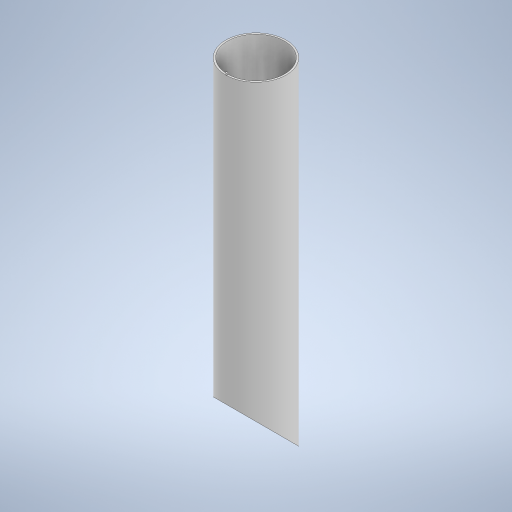
# Autodesk Inventor part: Feul_Intake
Saved by Autodesk Inventor 2024.3 (Build 283343000, 343)
## iProperties
Created: 2025-03-09
Part Number: Feul_Intake
Material: Generic
Document SubType Name: Modeling
Designer: ajclo
Density: 1 g/cm^3
Appearance: Default
Author: ajclo
Autodesk Inventor part; units mm, degrees
ref_plane "YZ Plane" through (0, 0, 0) normal (1, 0, 0) x (0, 1, 0)
ref_plane "XZ Plane" through (0, 0, 0) normal (0, 1, 0) x (-1, 0, 0)
ref_plane "XY Plane" through (0, 0, 0) normal (0, 0, 1) x (1, 0, 0)
sketch "Sketch1" plane through (0, 0, 0) normal (0, 1, 0) x (-1, 0, 0)
  circle A0 centre (0, 0) radius 35
  circle A1 centre (0, 0) radius 33
  dimension "d0" = 2
  dimension "d1" = 70
  constraints: 2 centre point, 2 coincident
  measures "d0" radial gap between concentric circles of A0 A1
  measures "d1" diameter of A0
extrude "Extrusion1" add sketch "Sketch1" along normal blind 400
sketch "Sketch2" plane through (0, 0, 0) normal (1, 0, 0) x (0, 1, 0)
  line L0 (0, -35) -> (0, 35) projected
  line L1 (0, -35) -> (70, 35)
  line L2 (0, 35) -> (400, 35) projected
  point P0 (0, 0)
  dimension "d4" = 70
  constraints: 2 end point, 1 point on line
  measures "d4" distance of L2.start L1.end
extrude "Extrusion2" cut sketch "Sketch2" along normal through all both and the other way through all
sketch "Sketch4" plane through (0, 400, 0) normal (0, 1, 0) x (1, 0, 0)
  circle A0 centre (0, -34) radius 1
  circle A1 centre (0, 0) radius 33 projected
  circle A2 centre (0, 0) radius 35 projected
  constraints: 2 tangent, 1 centre point
extrude "Extrusion4" add sketch "Sketch4" along normal blind 2 contours A0
body "Solid1"
